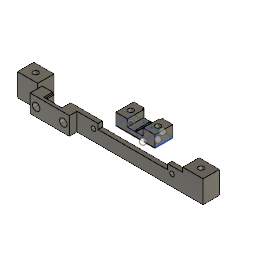
1-plug-mount v1 (Autodesk Fusion 360 design; units mm, degrees)
Autodesk Fusion 360 part; units mm, degrees
mesh "Mesh1" [no effect]
sketch "Body" plane through (0, 0, 0) normal (0, 0, 1) x (1, 0, 0) in component "PlugMountLarge"
  line L0 (-61.5, 8) -> (-48, 8)
  line L1 (-48, 8) -> (-48, 0)
  line L2 (-48, 0) -> (-40, 0)
  line L3 (-40, 0) -> (-40, -5.1)
  line L4 (-40, -5.1) -> (-30, -5.1)
  line L5 (-30, -5.1) -> (-30, 0)
  line L6 (-30, 0) -> (48, 0)
  line L7 (48, 0) -> (48, 8)
  line L8 (48, 8) -> (61.5, 8)
  line L9 (61.5, 8) -> (61.5, -3)
  line L10 (61.5, -3) -> (-22, -3)
  line L11 (-22, -3) -> (-22, -8)
  line L12 (-22, -8) -> (-48, -8)
  line L13 (-48, -8) -> (-48, -3)
  line L14 (-48, -3) -> (-61.5, -3)
  line L15 (-61.5, -3) -> (-61.5, 8)
  circle A0 centre (-54.75, 2.5) radius 1.75
  circle A1 centre (-54.75, 2.5) radius 2.5
  circle A2 centre (54.75, 2.5) radius 1.75
  circle A3 centre (54.75, 2.5) radius 2.5
  line L16 (-48, 0) -> (-48, -3)
  line L17 (-41, 0) -> (-41, -5.9)
  line L18 (-41, -5.9) -> (-29.06, -5.9)
  line L19 (-29.06, -5.9) -> (-29.06, 0)
  line L20 (48, 0) -> (48, -3)
  line L21 (-8, 0) -> (-8, -3)
  line L22 (38, 0) -> (38, -3)
  dimension "d1" = 11
  dimension "d2" = 13.5
  dimension "d3" = 78
  dimension "d4" = 8
  dimension "d5" = 13.5
  dimension "d6" = 26
  dimension "d7" = 5
  dimension "d8" = 8
  dimension "d9" = 10
  dimension "d10" = 5
  dimension "d11" = 3.5
  dimension "d12" = 5
  dimension "d13" = 3.5
  dimension "d14" = 5.9
  dimension "d15" = 5.1
  constraint horizontal L0
  constraint perpendicular L0 L1
  constraint perpendicular L1 L2
  constraint perpendicular L2 L3
  constraint perpendicular L3 L4
  constraint perpendicular L4 L5
  constraint perpendicular L5 L6
  constraint perpendicular L6 L7
  constraint perpendicular L7 L8
  constraint perpendicular L8 L9
  constraint perpendicular L9 L10
  constraint perpendicular L8 L11
  constraint perpendicular L11 L12
  constraint perpendicular L12 L13
  constraint perpendicular L13 L14
  constraint concentric A2 A3
  constraint perpendicular L14 L16
  constraint parallel L3 L17
  constraint perpendicular L17 L18
  constraint coincident L6 L19.end
  constraint perpendicular L6 L19
  constraint coincident L10 L20.end
  constraint perpendicular L10 L20
  constraint coincident L6 L21.start
  constraint coincident L10 L21.end
  constraint perpendicular L10 L21
  constraint coincident L6 L22.start
  constraint coincident L10 L22.end
  constraint perpendicular L10 L22
  measures "d1" distance of L0.start L14.end
  measures "d2" distance of L0.start L0.end
  measures "d3" distance of L5.end L6.end
  measures "d4" distance of L6.end L7.end
  measures "d5" distance of L7.end L8.end
  measures "d6" distance of L11.end L12.end
  measures "d7" distance of L12.end L13.end
  measures "d8" distance of L1.end L2.end
  measures "d9" distance of L3.end L4.end
  measures "d10" diameter of A1
  measures "d11" diameter of A0
  measures "d12" diameter of A3
  measures "d13" diameter of A2
  measures "d14" distance of L18.end L19.end
  measures "d15" distance of L4.end L5.end
extrude "Extrude2" add sketch "Body" along normal blind 12 contours L2 L6 L10 L11 L12 L13 L16 L17 L18 L19 L21 makes body 1 in component "PlugMountLarge"
extrude "Extrude1" add sketch "Body" along normal blind 11 contours L2 L3 L4 L5 L6 L17 L18 L19 bodies 1 in component "PlugMountLarge"
extrude "Extrude3" add sketch "Body" along normal blind 8.5 contours L6 L10 L21 L22 bodies 1 in component "PlugMountLarge"
extrude "Extrude4" add sketch "Body" along normal blind 15 contours L0 L1 L14 L15 L16 | A1 bodies 1 in component "PlugMountLarge"
extrude "Extrude5" cut sketch "Body" along normal blind 5 contours A1 bodies 1 in component "PlugMountLarge"
extrude "Extrude6" add sketch "Body" along normal blind 12 contours L6 L10 L20 L22 bodies 1 in component "PlugMountLarge"
extrude "Extrude7" add sketch "Body" along normal blind 15 contours L7 L8 L9 L10 L20 | A3 bodies 1 in component "PlugMountLarge"
extrude "Extrude8" cut sketch "Body" along normal blind 5 contours A3 bodies 1 in component "PlugMountLarge"
sketch "Holes1" plane through (0, -8, 0) normal (0, -1, 0) x (1, 0, 0) in component "PlugMountLarge"
  line L0 (-48, 0) -> (-22, 0)
  line L1 (-22, 0) -> (-22, 12)
  line L2 (-22, 12) -> (-48, 12)
  line L3 (-48, 12) -> (-48, 0)
  circle A0 centre (-44, 6) radius 1.75
  circle A1 centre (-44, 6) radius 2.5
  line L4 (-48, 6) -> (-22, 6) construction
  line L5 (-35, 12) -> (-35, 0) construction
  line L6 (-22, 6) -> (-48, 6) construction
  circle A2 centre (-26, 6) radius 2.5
  circle A3 centre (-26, 6) radius 1.75
  dimension "d32" = 3.5
  dimension "d33" = 5
  dimension "d34" = 6
  dimension "d35" = 4
  constraint concentric A0 A1
  constraint midpoint L3 L4.start
  constraint midpoint L1 L4.end
  constraint midpoint L2 L5.start
  constraint midpoint L0 L5.end
  constraint symmetric A0 L5 A3
  constraint symmetric A1 L5 A2
  constraint symmetric L4.start L5 L4.end
  constraint symmetric L4.end L5 L4.start
  measures "d32" diameter of A0
  measures "d33" diameter of A1
  measures "d34" distance of L2 A0.centre
  measures "d35" distance of L3 A0.centre
extrude "Extrude9" cut sketch "Holes1" against normal blind 8 contours A0 | A3 bodies 1 in component "PlugMountLarge"
extrude "Extrude10" cut sketch "Holes1" against normal blind 5 contours A1 | A2 bodies 1 in component "PlugMountLarge"
sketch "Holes2" plane through (0, -3, 0) normal (0, -1, 0) x (1, 0, 0) in component "PlugMountLarge"
  line L0 (-22, 0) -> (61.5, 0)
  line L1 (61.5, 0) -> (61.5, 15)
  line L2 (61.5, 15) -> (48, 15)
  line L3 (48, 15) -> (48, 12)
  line L4 (48, 12) -> (38, 12)
  line L5 (38, 12) -> (38, 8.5)
  line L6 (38, 8.5) -> (-8, 8.5)
  line L7 (-8, 8.5) -> (-8, 12)
  line L8 (-8, 12) -> (-22, 12)
  line L9 (-22, 12) -> (-22, 0)
  circle A0 centre (-11, 7.5) radius 1.5
  line L10 (15, 8.5) -> (15, 0) construction
  circle A1 centre (41, 7.5) radius 1.5
  line L11 (-22, 0) -> (-22, 12)
  dimension "d40" = 4.5
  dimension "d41" = 11
  constraint midpoint L6 L10.start
  constraint coincident L0 L10.end
  constraint symmetric A0 L10 A1
  measures "d40" distance of L8 A0.centre
  measures "d41" distance of A0.centre L11
extrude "Extrude11" cut sketch "Holes2" against normal blind 3 contours A0 | A1 bodies 1 in component "PlugMountLarge"
sketch "Sketch1" plane through (0, 0, 0) normal (0, 0, 1) x (1, 0, 0) in component "PlugMountSmall"
  line L0 (-13, 25.63) -> (13, 25.63)
  line L1 (13, 25.63) -> (13, 13.63)
  line L2 (13, 13.63) -> (-13, 13.63)
  line L3 (-13, 13.63) -> (-13, 25.63)
  line L4 (0, 25.63) -> (0, 13.63) construction
  line L5 (13, 19.63) -> (-13, 19.63) construction
  line L6 (-0.5, 24.33) -> (0.5, 24.33)
  line L7 (0.5, 24.33) -> (0.5, 14.33)
  line L8 (0.5, 14.33) -> (-0.5, 14.33)
  line L9 (-0.5, 14.33) -> (-0.5, 24.33)
  line L10 (-6, 25.63) -> (-6, 24.53)
  line L11 (-6, 24.53) -> (-5.2, 24.53)
  line L12 (-5.2, 24.53) -> (-5.2, 13.63)
  circle A0 centre (-9, 19.63) radius 1.75
  circle A1 centre (9, 19.63) radius 1.75
  line L13 (5.2, 24.53) -> (5.2, 13.63)
  line L14 (6, 24.53) -> (5.2, 24.53)
  line L15 (6, 25.63) -> (6, 24.53)
  line L16 (-5.2, 24.53) -> (5.2, 24.53)
  dimension "d44" = 26
  dimension "d45" = 12
  dimension "d46" = 10
  dimension "d47" = 1.3
  dimension "d48" = 1
  dimension "d49" = 0.5
  dimension "d50" = 3.5
  dimension "d51" = 0.8
  dimension "d52" = 1.1
  dimension "d53" = 7
  dimension "d54" = 4
  constraint horizontal L0
  constraint vertical L1
  constraint horizontal L2
  constraint vertical L3
  constraint midpoint L0 L4.start
  constraint midpoint L2 L4.end
  constraint midpoint L1 L5.start
  constraint midpoint L3 L5.end
  constraint horizontal L6
  constraint vertical L7
  constraint horizontal L8
  constraint vertical L9
  constraint coincident L0 L10.start
  constraint perpendicular L0 L10
  constraint perpendicular L10 L11
  constraint coincident L2 L12.end
  constraint perpendicular L2 L12
  constraint coincident L5 A0.centre
  constraint symmetric L4 L10.start L15.start
  constraint symmetric L4 L10.end L14.start
  constraint symmetric L4 L11.end L13.start
  constraint symmetric L4 L12.end L13.end
  constraint symmetric L4 A0 A1
  measures "d44" distance of L0.start L0.end
  measures "d45" distance of L0.end L1.end
  measures "d46" distance of L6.end L7.end
  measures "d47" distance of L0 L6
  measures "d48" distance of L6.start L6.end
  measures "d49" distance of L4 L7
  measures "d50" diameter of A0
  measures "d51" distance of L10.end L11.end
  measures "d52" distance of L10.start L10.end
  measures "d53" distance of L3 L10
  measures "d54" distance of L5.end A0.centre
extrude "Extrude1'" add sketch "Sketch1" along normal blind 3 separate body contours L2 L12 L13 L16 | L6 L7 L8 L9 makes body 2 in component "PlugMountSmall"
extrude "Extrude2'" add sketch "Sketch1" along normal blind 3.3 contours L6 L7 L8 L9 bodies 2 in component "PlugMountSmall"
extrude "Extrude3'" add sketch "Sketch1" along normal blind 2 contours L0 L10 L11 L14 L15 L16 bodies 2 in component "PlugMountSmall"
extrude "Extrude4'" add sketch "Sketch1" along normal blind 7.7 contours L0 L2 L3 L10 L11 L12 | L0 L1 L2 L13 L14 L15 bodies 2 in component "PlugMountSmall"
component "PlugMountLarge" placed x (1, 0, 0) y (0, 1, 0) z (0, 0, 1) at (0, 0, 0)
component "PlugMountSmall" placed x (1, 0, 0) y (0, 1, 0) z (0, 0, 1) at (0, 0, 0)
